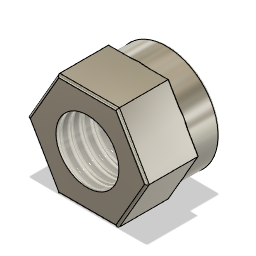
7.167.4471 - Ecrou HFR M10 (Autodesk Fusion 360 design; units mm, degrees)
Autodesk Fusion 360 part; units mm, degrees
sketch "Sketch1" plane through (0, 0, 0) normal (0, 0, 1) x (1, 0, 0)
  circle A0 centre (0, 0) radius 5
  circle A1 centre (0, 0) radius 7
  dimension "d1" = 10
  dimension "d2" = 2
  constraint coincident A0.centre A1.centre
  measures "d1" diameter of A0
extrude "Extrude1" add sketch "Sketch1" along normal blind 4
sketch "Sketch2" plane through (0, 0, 4) normal (0, 0, 1) x (1, 0, 0)
  circle A0 centre (0, 0) radius 5
  circle A1 centre (0, 0) radius 7
  line L0 (-4.0415, 7) -> (-8.0829, 0)
  line L1 (-8.0829, 0) -> (-4.0415, -7)
  line L2 (-4.0415, -7) -> (4.0415, -7)
  line L3 (4.0415, -7) -> (8.0829, 0)
  line L4 (8.0829, 0) -> (4.0415, 7)
  line L5 (4.0415, 7) -> (-4.0415, 7)
  circle A2 centre (0, 0) radius 5
  constraint coincident A0.centre A1.centre
extrude "Extrude2" add sketch "Sketch2" along normal blind 7
thread "Thread1" "ISO Metric profile 10.0 M10x1.5 6H" major diameter 10.198 minor diameter 8.526 pitch 1.5 angle 60 resizes the face on face at (4.9752, -0.4978, 3.6667)
fillet "Fillet1" radius 0.3 6 edges at (0, -7, 11) (-6.0622, -3.5, 11) (-6.0622, 3.5, 11) (0, 7, 11) (6.0622, 3.5, 11) (6.0622, -3.5, 11)
fillet "Fillet2" radius 0.1 12 edges at (-2.0207, -7, 4) (-5.0518, -5.25, 4) (-7.0725, -1.75, 4) (-7.0725, 1.75, 4) (-5.0518, 5.25, 4) (-2.0207, 7, 4) (2.0207, 7, 4) (5.0518, 5.25, 4) (7.0725, 1.75, 4) (7.0725, -1.75, 4) (5.0518, -5.25, 4) (2.0207, -7, 4)
fillet "Fillet3" radius 0.3 1 edges at (-6.5263, -2.5313, 0)
